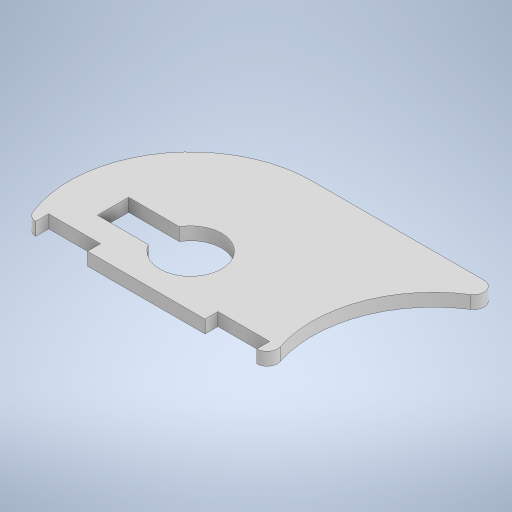
# Autodesk Inventor part: 皿
Saved by Autodesk Inventor 2024.1 (Build 281209000, 209)
## iProperties
Created: 2024-04-25
Part Number: 皿
Material: 一般
Document SubType Name: Modeling
Designer: hibik
Density: 1 g/cm^3
Appearance: 既定
Author: hibik
Autodesk Inventor part; units mm, degrees
ref_plane "YZ Plane" through (0, 0, 0) normal (1, 0, 0) x (0, 1, 0)
ref_plane "XZ Plane" through (0, 0, 0) normal (0, 1, 0) x (-1, 0, 0)
ref_plane "XY Plane" through (0, 0, 0) normal (0, 0, 1) x (1, 0, 0)
sketch "スケッチ1" plane through (0, 0, 0) normal (0, 1, 0) x (-1, 0, 0)
  circle A0 centre (0, 0) radius 6
  line L0 (0, 3) -> (15, 3)
  line L1 (15, 3) -> (15, -3)
  line L2 (15, -3) -> (0, -3)
  line L3 (0, -3) -> (0, 3) construction
  line L4 (23.5, 10) -> (-25.7338, 10)
  line L5 (-25.7338, 10) -> (-25.7338, -10) construction
  line L6 (-25.7338, -10) -> (23.5, -10)
  line L7 (23.5, -10) -> (23.5, 10) construction
  circle A1 centre (0, 0) radius 23.5
  circle A2 centre (-47, 0) radius 23.5
  line L8 (-23.5, 10) -> (-23.5, 0)
  line L9 (0, -23.5) -> (-47, -23.5)
  line L10 (0, 23.5) -> (-47, 23.5)
  point P0 (-25.7338, 0)
  point P1 (20.3516, -11.75)
  point P2 (-26.6484, -11.75)
  point P3 (5.1962, -3)
  point P4 (5.1962, 3)
  point P5 (21.2662, 10)
  point P6 (-21.2662, 10)
  dimension "d0" = 12
  dimension "d1" = 15
  dimension "d2" = 6
  dimension "d3" = 20
  dimension "d4" = 47
  dimension "d5" = 47
  dimension "d6" = 47
  constraints: 22 end point, 9 point on circle, 5 parallel, 3 centre point, 3 coincident, 3 horizontal, 3 tangent, 2 horizontal alignment, 2 midpoint, 2 perpendicular, 1 point on line, 1 vertical
  measures "d0" diameter of A0
  measures "d1" distance of L1.end L2.end
  measures "d2" distance of L0.end L1.end
  measures "d3" distance of L4.end L5.end
  measures "d4" diameter of A1
  measures "d5" diameter of A2
  measures "d6" distance of A2.centre point (0, 0)
extrude "押し出し1" add sketch "スケッチ1" along normal blind 2.5 contours L8 A2 L4 | L4 A1 L8 | L4 A1 L6 | A1 L6 A2 | A1 L9 A2 L6 | L6 A1
fillet "フィレット2" radius 2 3 edges at (47, 1.25, -23.5) (25.7338, 1.25, 10) (-21.2662, 1.25, 10)
sketch "スケッチ2" plane through (0, 2.5, 0) normal (0, 1, 0) x (1, 0, 0)
  line L0 (-19.9562, -10) -> (22.7874, -10) projected
  line L1 (-19.9562, -10) -> (22.7874, -10)
  line L2 (22.7874, -10) -> (22.7874, -7.5)
  line L3 (22.7874, -7.5) -> (-19.9562, -7.5)
  line L4 (-19.9562, -7.5) -> (-19.9562, -10)
  line L5 (-19.9562, -10) -> (-9.9562, -10)
  line L6 (-9.9562, -10) -> (-9.9562, -7.5)
  line L7 (-9.9562, -7.5) -> (-19.9562, -7.5)
  line L8 (-19.9562, -7.5) -> (-19.9562, -10)
  line L9 (22.7874, -10) -> (12.7874, -10)
  line L10 (12.7874, -10) -> (12.7874, -7.5)
  line L11 (12.7874, -7.5) -> (22.7874, -7.5)
  line L12 (22.7874, -7.5) -> (22.7874, -10)
  point P0 (0, 0)
  dimension "d13" = 2.5
  dimension "d14" = 10
  dimension "d15" = 10
  constraints: 24 end point, 6 parallel, 3 horizontal, 3 perpendicular, 2 point on line
  measures "d13" distance between parallel lines of L0 L3
  measures "d14" distance from line of L4 L6.end
  measures "d15" distance between parallel lines of L2 L10
extrude "押し出し2" cut sketch "スケッチ2" against normal through all contours L4 L3 L6 L0 | L10 L3 L2 L0
